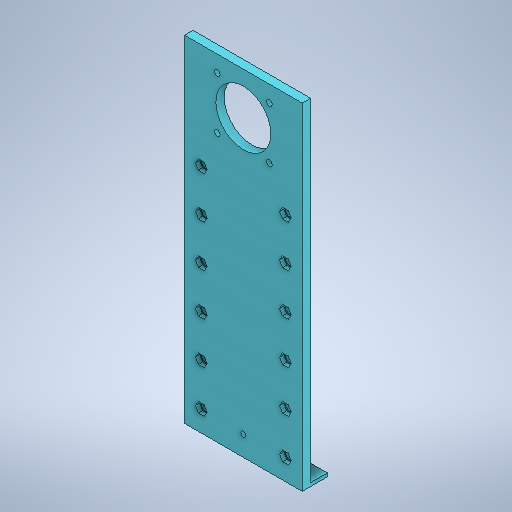
# Autodesk Inventor part: support_tete_prehension
Saved by Autodesk Inventor 2025.1 (Build 291241000, 241)
## iProperties
Created: 2025-03-10
Part Number: support_tete_prehension
Material: Générique
Document SubType Name: Modeling
Designer: felix
Density: 1 g/cm^3
Appearance: Vert turquoise
Author: felix
Autodesk Inventor part; units mm, degrees
ref_plane "YZ Plane" through (0, 0, 0) normal (1, 0, 0) x (0, 1, 0)
ref_plane "XZ Plane" through (0, 0, 0) normal (0, 1, 0) x (-1, 0, 0)
sketch "Esquisse1" plane through (0, 0, 0) normal (0, 0, 1) x (1, 0, 0)
  line L0 (0, 0) -> (70, 0)
  line L1 (70, 0) -> (70, 200)
  line L2 (70, 200) -> (0, 200)
  line L3 (0, 200) -> (0, 0)
  line L4 (35, 200) -> (35, 0) construction
  line L5 (10, 200) -> (10, 0) construction
  circle A0 centre (10, 12.5) radius 2.5
  circle A1 centre (10, 37.5) radius 2.5
  circle A2 centre (10, 62.5) radius 2.5
  circle A3 centre (10, 87.5) radius 2.5
  circle A4 centre (10, 112.5) radius 2.5
  circle A5 centre (10, 137.5) radius 2.5
  circle A6 centre (60, 12.5) radius 2.5
  circle A7 centre (60, 37.5) radius 2.5
  circle A8 centre (60, 62.5) radius 2.5
  circle A9 centre (60, 87.5) radius 2.5
  circle A10 centre (60, 112.5) radius 2.5
  circle A11 centre (60, 137.5) radius 2.5
  circle A12 centre (50.5, 190.3544) radius 1.7
  circle A13 centre (50.5, 159.3544) radius 1.7
  circle A14 centre (19.5, 159.3544) radius 1.7
  circle A15 centre (19.5, 190.3544) radius 1.7
  circle A16 centre (35, 174.8544) radius 21.9203 construction
  circle A17 centre (35, 174.8544) radius 16.3737
  point P0 (35, 0)
  dimension "d0" = 200
  dimension "d3" = 70
  dimension "d16" = 35
  dimension "d18" = 15.5
  dimension "d22" = 31
  dimension "d25" = 31
  dimension "d70" = 12.5
  dimension "d73" = 25
  dimension "d76" = 50
  dimension "d79" = 10
  dimension "d80" = 10
  dimension "d110" = 3.4
  dimension "d111" = 3.4
  dimension "d112" = 3.4
  dimension "d113" = 3.4
  constraints: 18 centre point, 12 end point, 5 coincident, 4 midpoint, 3 horizontal, 3 perpendicular, 3 point on circle, 3 point on line, 2 parallel, 2 vertical, 26 other
  measures "d0" distance of L0.end L1.end
  measures "d3" distance of L1.end L2.end
  measures "d16" distance of point (35, 0) L0.start
  measures "d18" distance from line of L4 point (19.5, 190.354)
  measures "d22" distance of point (19.5, 190.354) point (50.5, 190.354)
  measures "d25" distance of point (19.5, 190.354) point (19.5, 159.354)
  measures "d70" distance of L5.end A0.centre
  measures "d73" distance of A0.centre A1.centre
  measures "d76" distance of A0.centre A6.centre
  measures "d79" distance from line of L3 A0.centre
  measures "d80" distance from line of L1 A6.centre
  measures "d110" diameter of A12
  measures "d111" diameter of A13
  measures "d112" diameter of A15
  measures "d113" diameter of A14
extrude "Extrusion1" add sketch "Esquisse1" along normal blind 5
sketch "Esquisse4" plane through (0, 0, 5) normal (0, 0, 1) x (1, 0, 0)
  circle A0 centre (10, 12.5) radius 2.5 projected
  line L0 (11.7955, 15.4624) -> (13.4633, 12.4262)
  line L1 (13.4633, 12.4262) -> (11.6678, 9.4638)
  line L2 (11.6678, 9.4638) -> (8.2045, 9.5376)
  line L3 (8.2045, 9.5376) -> (6.5367, 12.5738)
  line L4 (6.5367, 12.5738) -> (8.3322, 15.5362)
  line L5 (8.3322, 15.5362) -> (11.7955, 15.4624)
  point P0 (0, 0)
  point P1 (12.6294, 13.9443)
  dimension "d45" = 6
  constraints: 12 end point, 1 coincident, 1 midpoint, 13 other
  measures "d45" distance from line of L3 point (12.629, 13.944)
extrude "Extrusion3" cut sketch "Esquisse4" against normal blind 2.5
pattern_linear "Réseau rectangulaire1" count 6 spacing 25 along (0, 1, 0) of "Extrusion3"
ref_plane "Plan de construction1" through (35, 0, 0) normal (-1, 0, 0) x (0, 0, 1)
mirror "Mise en miroir1" about plane through (35, 0, 0) normal (-1, 0, 0) of "Extrusion3", "Réseau rectangulaire1"
sketch "Esquisse7" plane through (0, 0, 5) normal (0, 0, 1) x (1, 0, 0)
  line L0 (70, 0) -> (70, 200) projected
  line L1 (0, 0) -> (70, 0)
  line L2 (0, 0) -> (70, 0)
  line L3 (70, 0) -> (70, 2)
  line L4 (70, 2) -> (0, 2)
  line L5 (0, 2) -> (0, 0)
  dimension "d81" = 70
  dimension "d82" = 2
  constraints: 10 end point, 2 horizontal, 2 parallel, 1 perpendicular, 1 point on line
  measures "d81" distance of L1.start L0.start
  measures "d82" distance of L4.end L1.start
extrude "Extrusion5" add sketch "Esquisse7" against normal blind 15
sketch "Esquisse9" plane through (0, 0, 0) normal (0, 0, -1) x (-1, 0, 0)
  line L0 (-70, 0) -> (-70, 200) construction
  line L1 (0, 0) -> (-70, 0) construction
  point P0 (-35, 12)
  dimension "d95" = 70
  dimension "d96" = 12
  dimension "d97" = 35
  constraints: 2 end point, 1 horizontal
  measures "d95" distance of L1.start L0.start
  measures "d96" distance from line of L1 point (-35, 12)
  measures "d97" distance from line of L0 point (-35, 12)
hole "Perçage4" at (35, 12, 0) direction (0, 0, 1) diameter 3.1 depth 5 tip angle 118 clearance for "Vis d'assemblage à six pans creux" size "M3" standard "Profil M métrique ANSI"
sketch "Esquisse10" plane through (0, 0, 0) normal (0, 0, -1) x (-1, 0, 0)
  circle A0 centre (-35, 12) radius 1.55 projected
  circle A1 centre (-35, 12) radius 2.5
  circle A2 centre (-35, 12) radius 1.6
  point P0 (0, 0)
  dimension "d105" = 3.2
  dimension "d106" = 5
  constraints: 2 centre point, 2 coincident
  measures "d105" diameter of A2
  measures "d106" diameter of A1
extrude "Extrusion6" add sketch "Esquisse10" along normal blind 1.5 contours A1
fillet "Congé4" radius 1.5 1 edges at (37.5, 12, 0)
equation "\"d111\" = d110"
equation "\"d112\" = d110"
equation "\"d113\" = d110"
equation "\"d97\" = 0.5 * d95"
